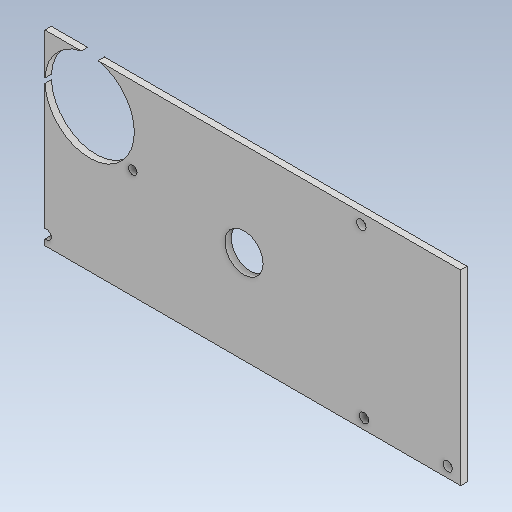
# Autodesk Inventor part: Part7
Saved by Autodesk Inventor 2020.2 (Build 242310000, 310)
## iProperties
Created: 2022-11-14
Part Number: Part7
Material: 一般
Document SubType Name: Modeling
Designer: Administrator
Density: 1 g/cm^3
Appearance: 既定
Author: Administrator
Autodesk Inventor part; units mm, degrees
ref_plane "YZ Plane" through (0, 0, 0) normal (1, 0, 0) x (0, 1, 0)
ref_plane "XZ Plane" through (0, 0, 0) normal (0, 1, 0) x (-1, 0, 0)
ref_plane "XY Plane" through (0, 0, 0) normal (0, 0, 1) x (1, 0, 0)
sketch "スケッチ1" plane through (0, 0, 0) normal (0, 0, 1) x (1, 0, 0)
  line L0 (84.1565, -23.7) -> (79.5065, -23.7) projected
  line L1 (79.5065, -23.7) -> (79.5065, -42.5843) projected
  line L2 (79.5065, -42.5843) -> (81.2722, -44.35) projected
  line L3 (81.2722, -44.35) -> (110.4408, -44.35) projected
  line L4 (110.4408, -44.35) -> (112.2065, -42.5843) projected
  line L5 (112.2065, -42.5843) -> (112.2065, -23.7) projected
  line L6 (112.2065, -23.7) -> (107.5565, -23.7) projected
  arc A0 (107.0565, -23.2) -> (107.5565, -23.7) centre (107.5565, -23.2) ccw projected
  line L7 (107.0565, -23.2) -> (107.0565, -21.9243) projected
  arc A1 (107.0565, -21.9243) -> (107.0272, -21.8536) centre (106.9565, -21.9243) ccw projected
  line L8 (107.0272, -21.8536) -> (103.903, -18.7293) projected
  arc A2 (103.903, -18.7293) -> (103.8323, -18.7) centre (103.8323, -18.8) ccw projected
  line L9 (103.8323, -18.7) -> (87.8808, -18.7) projected
  arc A3 (87.8808, -18.7) -> (87.8101, -18.7293) centre (87.8808, -18.8) ccw projected
  line L10 (87.8101, -18.7293) -> (84.6858, -21.8536) projected
  arc A4 (84.6858, -21.8536) -> (84.6565, -21.9243) centre (84.7565, -21.9243) ccw projected
  line L11 (84.6565, -21.9243) -> (84.6565, -23.2) projected
  arc A5 (84.1565, -23.7) -> (84.6565, -23.2) centre (84.1565, -23.2) ccw projected
  circle A6 centre (109.3565, -41.5) radius 2.4 projected
  circle A7 centre (82.3565, -41.5) radius 2.4 projected
  line L12 (112.6065, -10.3) -> (112.6065, 11.75) projected
  line L13 (112.6065, -42.75) -> (112.6065, -23.5) projected
  line L14 (110.6065, 13.75) -> (99.8565, 13.75) projected
  line L15 (81.1065, -44.75) -> (110.6065, -44.75) projected
  circle A8 centre (45.5709, -15.5) radius 5 projected
  line L16 (11.9799, 13.75) -> (-17.5201, 13.75) projected
  line L17 (11.8143, 13.35) -> (-17.3544, 13.35) projected
  line L18 (-17.3544, 13.35) -> (-19.1201, 11.5843) projected
  line L19 (-19.1201, 11.5843) -> (-19.1201, -42.5843) projected
  line L20 (-19.1201, -42.5843) -> (-17.3544, -44.35) projected
  line L21 (-17.3544, -44.35) -> (11.8143, -44.35) projected
  line L22 (11.8143, -44.35) -> (13.5799, -42.5843) projected
  line L23 (13.5799, -42.5843) -> (13.5799, 11.5843) projected
  line L24 (13.5799, 11.5843) -> (11.8143, 13.35) projected
  circle A9 centre (-16.2701, 10.5) radius 2.4 projected
  circle A10 centre (10.7299, -41.5) radius 2.4 projected
  circle A11 centre (-16.2701, -41.5) radius 2.4 projected
  circle A12 centre (10.7299, -10.5) radius 1.35 projected
  circle A13 centre (-16.2701, -10.5) radius 1.35 projected
  circle A14 centre (10.7299, 10.5) radius 2.4 projected
  circle A15 centre (-2.7701, 0) radius 13 projected
  circle A16 centre (10.7299, -41.5) radius 1.3 projected
  circle A17 centre (10.7299, 10.5) radius 1.3 projected
  circle A18 centre (-16.2701, 10.5) radius 1.3 projected
  circle A19 centre (-16.2701, -41.5) radius 1.3 projected
  line L25 (-17.5201, -44.75) -> (11.9799, -44.75) projected
  line L26 (-19.5201, 11.75) -> (-19.5201, -42.75) projected
  circle A20 centre (109.3565, 10.5) radius 2.4 projected
  circle A21 centre (109.3565, 10.5) radius 1.3 projected
  circle A22 centre (109.3565, -41.5) radius 1.3 projected
  circle A23 centre (82.3565, -41.5) radius 1.3 projected
  circle A24 centre (82.3565, 10.5) radius 1.3 projected
  circle A25 centre (82.3565, 10.5) radius 2.4 projected
  line L27 (79.1065, 11.75) -> (79.1065, -10.3) projected
  line L28 (-16.75, 13.75) -> (113.432, 13.75)
  line L29 (113.432, 13.75) -> (113.432, -44.75)
  line L30 (113.432, -44.75) -> (-16.75, -44.75)
  line L31 (-16.75, -44.75) -> (-16.75, 13.75)
  circle A26 centre (-2.7701, 0) radius 14
  circle A27 centre (10.7299, 10.5) radius 1.5
  circle A28 centre (-16.2701, 10.5) radius 1.5
  circle A29 centre (10.7299, -41.5) radius 1.5
  circle A30 centre (-16.2701, -41.5) radius 1.5
  circle A31 centre (109.3565, 10.5) radius 1.5
  circle A32 centre (82.3565, 10.5) radius 1.5
  circle A33 centre (109.3565, -41.5) radius 1.5
  circle A34 centre (83.182, -41.5) radius 1.5
  circle A35 centre (45.5709, -15.5) radius 6
  point P0 (0, 0)
  point P1 (-5.404, 13.75)
  point P2 (-16.75, 13.75)
  point P3 (-16.75, 11.75)
  point P4 (-16.75, 0.16)
  point P5 (-16.75, -44.75)
  point P6 (113.432, -42.75)
  point P7 (113.432, -23.5)
  point P8 (113.432, -32.66)
  point P9 (113.432, 11.75)
  point P10 (-0.1361, 13.75)
  point P11 (-0.1361, 13.75)
  point P12 (-5.404, 13.75)
  point P13 (-9.4326, 13.75)
  dimension "d0" = 28
  dimension "d1" = 3
  dimension "d2" = 3
  dimension "d3" = 3
  dimension "d4" = 3
  dimension "d5" = 3
  dimension "d6" = 3
  dimension "d7" = 3
  dimension "d8" = 3
  dimension "d9" = 12
  constraints: 10 centre point, 9 coincident, 8 end point, 2 parallel, 1 horizontal, 1 perpendicular
  measures "d0" diameter of A26
  measures "d1" diameter of A27
  measures "d2" diameter of A28
  measures "d3" diameter of A29
  measures "d4" diameter of A30
  measures "d5" diameter of A31
  measures "d6" diameter of A32
  measures "d7" diameter of A33
  measures "d8" diameter of A34
  measures "d9" diameter of A35
extrude "押し出し1" add sketch "スケッチ1" along normal blind 2 contours A5 L11 A4 L10 A3 L9 A2 L8 A1 L7 A0 L6 L5 L4 L3 L2 L1 L0 | A6 | A7 | L28 L29 L30 L15 L25 L31 L21 L22 L23 L24 L17 A26 L16 L14 | A26 L17 L31 L16 | L17 L24 L23 L22 L21 L31 A11 A13 A26 | A26 L31 A9 L17 | A9 L31 A28 | A13 L31 | A28 L31 A18 | L31 A30 A11 | A18 L31 | A10 | A14 | A16 | A17 | A20 | A21 | A34 A23 | A25 | A27 | A29 | A31 picked at (-14.1896, 10.3242) picked at (-15.7377, -10.5576) picked at (-14.8507, 10.3826) picked at (-14.1896, -41.6758) picked at (-15.9577, 10.2068) picked at (81.4802, -41.5)
